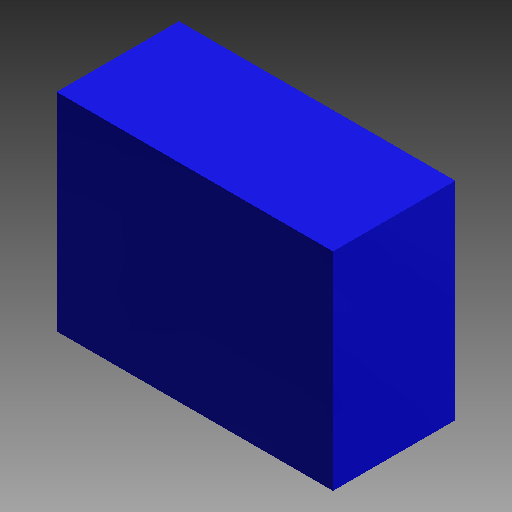
# Autodesk Inventor part: 1uF
Saved by Autodesk Inventor 2018.2 (Build 222227000, 227)
## iProperties
Part Number: 1uF
Material: Generic
Document SubType Name: Modeling
Designer: autocad
Appearance: C0805, 1uF
Author: autocad
Autodesk Inventor part; units mm, degrees
ref_plane "YZ Plane" through (0, 0, 0) normal (1, 0, 0) x (0, 1, 0)
ref_plane "XZ Plane" through (0, 0, 0) normal (0, 1, 0) x (-1, 0, 0)
ref_plane "XY Plane" through (0, 0, 0) normal (0, 0, 1) x (1, 0, 0)
sketch "C0805, 1uF_69" plane through (0, 0, 0) normal (0, 0, 1) x (1, 0, 0)
  line L0 (1.016, 0.762) -> (1.016, -0.762)
  line L1 (1.016, -0.762) -> (-1.016, -0.762)
  line L2 (-1.016, -0.762) -> (-1.016, 0.762)
  line L3 (-1.016, 0.762) -> (1.016, 0.762)
  constraints: 8 end point
extrude "Extrusion1" add sketch "C0805, 1uF_69" along normal blind 0.9
body "Solid1"
